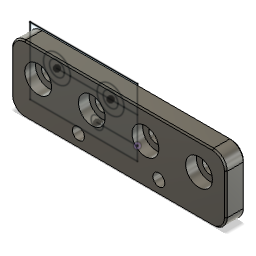
JKK60_RailTo2080ProfileAdapter v5 (Autodesk Fusion 360 design; units mm, degrees)
Autodesk Fusion 360 part; units mm, degrees
note: some values were not read from the file. Set by a fixed rule: which sketch regions a step uses.
sketch "Skizze1" plane through (0, 0, 0) normal (0, 0, 1) x (1, 0, 0)
  circle A0 centre (-15, 0) radius 2.25
  circle A1 centre (-30, 10) radius 2.75
  line L0 (-40, 20) -> (0, 20)
  line L1 (0, 20) -> (0, -5)
  line L2 (0, -5) -> (-40, -5)
  line L3 (-40, -5) -> (-40, 20)
  circle A2 centre (-10, 10) radius 2.75
  line L4 (-30, 10) -> (0, 10)
  circle A3 centre (-10, 10) radius 5
  circle A4 centre (-30, 10) radius 5
  line L5 (-15, 0) -> (0, 0)
  dimension "d1" = 4.5
  dimension "d2" = 15
  dimension "d4" = 5.5
  dimension "d5" = 40
  dimension "d16" = 30
  dimension "d17" = 20
  dimension "d18" = 10
  dimension "d19" = 10
  dimension "d20" = 10
  dimension "d21" = 5
  constraint horizontal L0
  constraint vertical L1
  constraint horizontal L2
  constraint vertical L3
  constraint coincident L5.end L1
  constraint coincident A1.centre L4.start
  constraint coincident L1 L4.end
  constraint perpendicular L1 L4
  constraint coincident A2.centre L4
  constraint equal A1 A2
  constraint concentric A2 A3
  constraint concentric A1 A4
  constraint equal A3 A4
  constraint coincident A0.centre L5.start
  constraint coincident L5.end origin
  constraint perpendicular L1 L5
  measures "d1" diameter of A0
  measures "d2" distance of L5.end A0.centre
  measures "d4" diameter of A1
  measures "d5" distance of L0.start L0.end
  measures "d16" distance of A1.centre L4.end
  measures "d17" horizontal distance of A1.centre A2.centre
  measures "d18" diameter of A4
  measures "d19" vertical distance of A0.centre A2.centre
  measures "d20" distance of L0 A1.centre
  measures "d21" distance of A0.centre L2
extrude "Extrusion1" add sketch "Skizze1" along normal blind 7 contours L0 L1 L2 L3
extrude "Extrusion2" add sketch "Skizze1" along normal blind 3 contours A2 L4 A3 | A2 L4 A3 | A4
fillet "Abrundung1" radius 5 2 edges at (-40, 20, 3.5) (-40, -5, 3.5)
mirror "Spiegeln1" about plane through (0, 20, 0) normal (1, 0, 0) of bodies 1 merged
chamfer "Fase1" distance 0.5 angle 45 16 edges at (0, 20, 7) (38.5355, 18.5355, 7) (40, 7.5, 7) (38.5355, -3.5355, 7) (0, -5, 7) (-38.5355, -3.5355, 7) (-40, 7.5, 7) (-38.5355, 18.5355, 7) (0, -5, 0) (-38.5355, -3.5355, 0) (-40, 7.5, 0) (-38.5355, 18.5355, 0) (0, 20, 0) (38.5355, 18.5355, 0) (40, 7.5, 0) (38.5355, -3.5355, 0)
equation "d2 = ( 30 / 2 ) * 1 mm"
equation "d5 = ( 80 / 2 ) * 1 mm"
equation "d16 = ( 80 / 2 ) * 1 mm - 10 mm"
